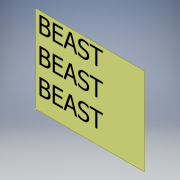
# Autodesk Inventor part: picture
Saved by Autodesk Inventor 2016 (Build 200138000, 138)
## iProperties
Created: 2016-11-17
Part Number: picture
Material: Generic
Document SubType Name: Modeling
Designer: 17kressc
Density: 1 g/cm^3
Appearance: Satin - Lemon Chiffon
Author: 17kressc
Autodesk Inventor part; units mm, degrees
ref_plane "YZ Plane" through (0, 0, 0) normal (1, 0, 0) x (0, 1, 0)
ref_plane "XZ Plane" through (0, 0, 0) normal (0, 1, 0) x (-1, 0, 0)
ref_plane "XY Plane" through (0, 0, 0) normal (0, 0, 1) x (1, 0, 0)
sketch "Sketch1" plane through (0, 0, 0) normal (0, 0, 1) x (1, 0, 0)
  point P0 (0, 0)
sketch "Sketch2" plane through (0, 0, 0) normal (0, 0, 1) x (1, 0, 0)
  line L0 (0, 0) -> (254, 0)
  line L1 (254, 0) -> (254, 203.2)
  line L2 (254, 203.2) -> (0, 203.2)
  line L3 (0, 203.2) -> (0, 0)
  dimension "d0" = 254
  dimension "d1" = 203.2
  constraints: 8 end point, 2 parallel, 1 horizontal, 1 perpendicular
  measures "d0" distance of L2.end L1.end
  measures "d1" distance of L1.end L0.end
extrude "Extrusion1" add sketch "Sketch2" along normal blind 0.0254
sketch "Sketch3" plane through (0, 0, 0.0254) normal (0, 0, 1) x (1, 0, 0)
  line L0 (5.5324, 195.9036) -> (248.5473, 195.9036) construction
  line L1 (248.5473, 195.9036) -> (248.5473, 8.8207) construction
  line L2 (248.5473, 8.8207) -> (5.5324, 8.8207) construction
  line L3 (5.5324, 8.8207) -> (5.5324, 195.9036) construction
  point P0 (0, 0)
  constraints: 2 other
body "Solid1"
